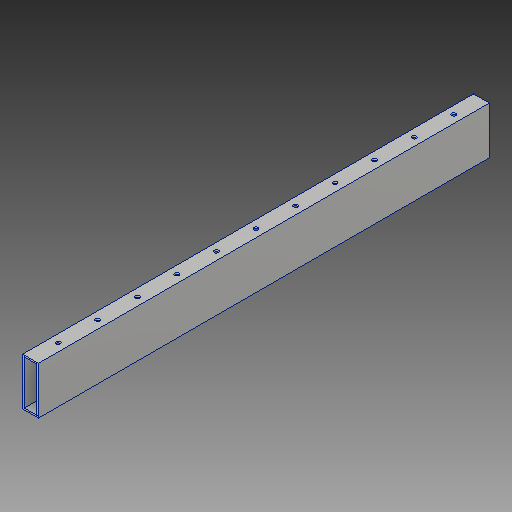
# Autodesk Inventor part: Back Extrusion
Saved by Autodesk Inventor 2019.4 (Build 234330000, 330)
## iProperties
Created: 2020-01-05
Part Number: Back Extrusion
Material: Aluminum 6061
Document SubType Name: Modeling
Designer: Mark
Mass: 466.445 g
Surface Area: 1737.45 cm^2
Volume: 172.757 cm^3
Density: 2.7 g/cm^3
Appearance: Aluminum - Flat
Author: Mark
Autodesk Inventor part; units mm, degrees
ref_plane "YZ Plane" through (0, 0, 0) normal (1, 0, 0) x (0, 1, 0)
ref_plane "XZ Plane" through (0, 0, 0) normal (0, 1, 0) x (-1, 0, 0)
ref_plane "XY Plane" through (0, 0, 0) normal (0, 0, 1) x (1, 0, 0)
sketch "Sketch1" plane through (0, 0, 0) normal (0, 0, 1) x (1, 0, 0)
  line L0 (-10, -30) -> (10, -30)
  line L1 (10, -30) -> (10, 30)
  line L2 (10, 30) -> (-10, 30)
  line L3 (-10, 30) -> (-10, -30)
  line L4 (-10, -30) -> (10, 30) construction
  line L5 (10, -30) -> (-10, 30) construction
  line L6 (8, -28) -> (-8, -28)
  line L7 (-8, -28) -> (-8, 28)
  line L8 (-8, 28) -> (8, 28)
  line L9 (8, 28) -> (8, -28)
  line L10 (8, -28) -> (-8, 28) construction
  line L11 (-8, -28) -> (8, 28) construction
  point P0 (0, 0)
  dimension "d0" = 20
  dimension "d1" = 60
  dimension "d2" = 16
  dimension "d3" = 56
  constraints: 24 end point, 4 midpoint, 4 parallel, 2 horizontal, 2 perpendicular
  measures "d0" distance of L2.end L1.end
  measures "d1" distance of L1.end L0.end
  measures "d2" distance of L7.end L8.end
  measures "d3" distance of L6.end L7.end
extrude "Extrusion1" add sketch "Sketch1" along normal blind 570
sketch "Sketch2" plane through (-10, 30, 0) normal (0, 1, 0) x (1, 0, 0)
  circle A0 centre (10, -535) radius 2.75
  line L0 (0, 0) -> (0, -570) projected
  circle A1 centre (10, -485) radius 2.75
  circle A2 centre (10, -435) radius 2.75
  circle A3 centre (10, -385) radius 2.75
  circle A4 centre (10, -335) radius 2.75
  circle A5 centre (10, -285) radius 2.75
  circle A6 centre (10, -235) radius 2.75
  circle A7 centre (10, -185) radius 2.75
  circle A8 centre (10, -135) radius 2.75
  circle A9 centre (10, -85) radius 2.75
  circle A10 centre (10, -35) radius 2.75
  circle A11 centre (10, 15) radius 2.75
  circle A12 centre (10, 65) radius 2.75
  circle A13 centre (10, 115) radius 2.75
  circle A14 centre (10, 165) radius 2.75
  line L1 (20, -570) -> (0, -570) projected
  point P0 (10, 0)
  dimension "d6" = 5.5
  dimension "d7" = 10
  dimension "d10" = 50
  dimension "d15" = 35
  constraints: 15 centre point, 1 vertical, 28 other
  measures "d6" diameter of A0
  measures "d7" distance from line of L0 A0.centre
  measures "d10" distance of A0.centre A1.centre
  measures "d15" distance from line of L1 A0.centre
extrude "Extrusion2" cut sketch "Sketch2" against normal blind 6 contours A0 | A1 | A2 | A3 | A4 | A5 | A6 | A7 | A8 | A9 | A10
body "Solid1"
